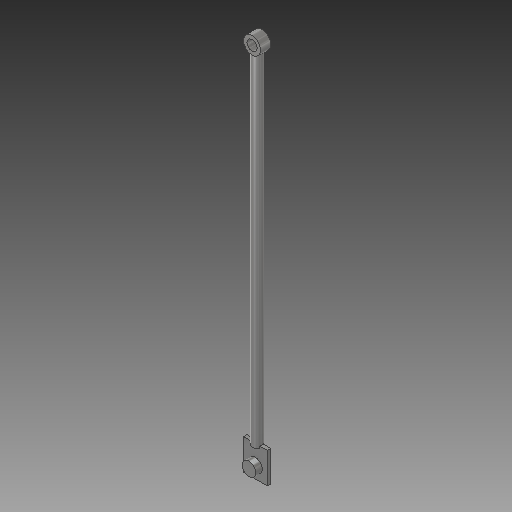
# Autodesk Inventor part: 101-05
Saved by Autodesk Inventor 2019 (Build 230136000, 136)
## iProperties
Company: Autodesk Inc.
Created: 2017-03-14
Part Number: 101-05
Material: Aluminum 6061
Document SubType Name: Modeling
Designer: Autodesk Inc.
Density: 2.7 g/cm^3
Appearance: Aluminum - Anodized Glossy (Grey)
Mass: 2.02858 g
Surface Area: 11.6499 cm^2
Volume: 0.751327 cm^3
Author: Inventor
Autodesk Inventor part; units mm, degrees
ref_plane "YZ Plane" through (0, 0, 0) normal (1, 0, 0) x (0, 1, 0)
sketch "Sketch1" plane through (0, 0, 0) normal (0, 1, 0) x (-1, 0, 0)
  circle A0 centre (0, 0) radius 1.4
  dimension "d0" = 2.8
  constraints: 1 centre point, 1 coincident
  measures "d0" diameter of A0
extrude "Extrusion1" add sketch "Sketch1" along normal blind 100
ref_plane "Work Plane1" through (0, 99.5, 0) normal (0, 1, 0) x (1, 0, 0)
sketch "Sketch2" plane through (0, 99.5, 0) normal (0, 1, 0) x (1, 0, 0)
  line L0 (0, 0) -> (0, -1.5)
  line L1 (0, 0) -> (0, 1.5)
  dimension "d4" = 1.5
  dimension "d5" = 1.5
  constraints: 4 end point, 2 vertical
  measures "d4" distance of L0.start L0.end
  measures "d5" distance of L0.start L1.end
sketch "Sketch3" plane through (0, 0, 0) normal (1, 0, 0) x (0, 1, 0)
  line L0 (99.5, 0) -> (99.5, 1.5) projected
  line L1 (99.5, 0) -> (99.5, -1.5) projected
  line L2 (99.5, 1.5) -> (100.5, 1.5)
  line L3 (100.5, 1.5) -> (100.5, -1.5)
  line L4 (100.5, -1.5) -> (99.5, -1.5)
  line L5 (102, 1.659) -> (102, -3.2084)
  point P0 (0, 0)
  dimension "d6" = 1
  dimension "d7" = 2.5
  constraints: 8 end point, 2 perpendicular, 1 horizontal, 1 vertical
  measures "d6" distance of L0.end L2.end
  measures "d7" distance between parallel lines of L0 L5
revolve "Revolution1" add sketch "Sketch3" angle 360 about axis through (0, 102, 1.659) along (0, 0, -1)
ref_plane "Work Plane2" through (0, 0.5, 0) normal (0, -1, 0) x (1, 0, 0)
sketch "Sketch4" plane through (0, 0.5, 0) normal (0, -1, 0) x (1, 0, 0)
  line L0 (0, 0) -> (0, -2.1121)
  line L1 (3.5, -0.5) -> (3.5, 0.5)
  line L2 (3.5, 0.5) -> (0, 0.5)
  line L3 (3.5, -0.5) -> (0, -0.5)
  line L4 (-3.5, -0.5) -> (-3.5, 0.5)
  line L5 (-3.5, 0.5) -> (0, 0.5)
  line L6 (-3.5, -0.5) -> (0, -0.5)
  dimension "d12" = 3.5
  dimension "d13" = 1
  constraints: 14 end point, 2 point on line, 2 symmetric about line, 2 vertical, 1 horizontal, 1 perpendicular, 1 other
  measures "d12" distance of L4.end L2.end
  measures "d13" distance of L4.start L4.end
extrude "Extrusion2" add sketch "Sketch4" along normal blind 9
sketch "Sketch5" plane through (3.5, 0.5, -0.5) normal (0, 0, -1) x (-1, 0, 0)
  line L0 (3.5, -0.5) -> (3.5, -9)
  line L1 (7, -9) -> (0, -9) projected
  line L2 (3.5, -9) -> (3.5, -5.5)
  line L3 (3.5, -9) -> (3.5, -9.0551)
  circle A0 centre (3.5, -5.5) radius 2
  dimension "d16" = 3.5
  dimension "d17" = 4
  constraints: 6 end point, 2 coincident, 2 midpoint, 2 vertical, 1 centre point, 1 point on line
  measures "d16" distance of L0.end L2.end
  measures "d17" diameter of A0
extrude "Extrusion3" add sketch "Sketch5" along normal blind 1.2
sketch "Sketch6" plane through (-3.5, 0.5, 0.5) normal (0, 0, 1) x (1, 0, 0)
  circle A0 centre (3.5, -5.5) radius 2 projected
  point P0 (3.5, -0.5)
extrude "Extrusion4" add sketch "Sketch6" along normal blind 1.9
body "Solid1"
